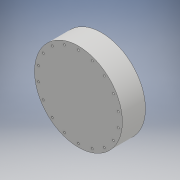
# Autodesk Inventor part: Korbbogenboden
Saved by Autodesk Inventor 2017 (Build 210142000, 142)
## iProperties
Created: 2019-06-21
Part Number: Korbbogenboden
Material: Generic
Document SubType Name: Modeling
Designer: Ole Simmering
Density: 1 g/cm^3
Appearance: Default
Author: Ole Simmering
Autodesk Inventor part; units mm, degrees
ref_plane "YZ Plane" through (0, 0, 0) normal (1, 0, 0) x (0, 1, 0)
ref_plane "XZ Plane" through (0, 0, 0) normal (0, 1, 0) x (-1, 0, 0)
ref_plane "XY Plane" through (0, 0, 0) normal (0, 0, 1) x (1, 0, 0)
sketch "Sketch1" plane through (0, 0, 0) normal (0, 0, 1) x (1, 0, 0)
  line L0 (0, 26.4298) -> (0, -158.7692) construction
  line L1 (144, 0) -> (144, -25)
  arc A0 (125.4705, -49.1481) -> (144, -25) centre (119, -25) ccw
  arc A1 (0, -66.1697) -> (125.4705, -49.1481) centre (-3.939, 433.8148) ccw
  line L2 (144, 0) -> (190, 0)
  line L3 (190, 0) -> (190, -100)
  line L4 (190, -100) -> (0, -100)
  line L5 (144, -25) -> (119, -25) construction
  line L6 (125.4705, -49.1481) -> (119, -25) construction
  line L7 (0, -66.1697) -> (0, -100)
  point P0 (0, 0)
  dimension "d0" = 288
  dimension "d1" = 380
  dimension "d2" = 100
  dimension "d3" = 25
  dimension "d4" = 500
  dimension "d5" = 25
  dimension "d6" = 75
  constraints: 16 end point, 4 point on circle, 3 horizontal, 3 point on line, 2 centre point, 2 tangent, 2 vertical, 1 collinear, 1 midpoint, 1 perpendicular
  measures "d0" diameter of L1 L0
  measures "d1" diameter of L3 L0
  measures "d2" distance of L2.end L3.end
  measures "d3" radius of A0
  measures "d4" radius of A1
  measures "d5" distance of L1.start L1.end
  measures "d6" angle of L6 L5
revolve "Revolution1" add sketch "Sketch1" angle 360 about axis through (0, 26.4298, 0) along (0, -1, 0)
sketch "Sketch2" plane through (0, 0, 0) normal (0, 1, 0) x (1, 0, 0)
  point P0 (0, 0)
  point P1 (0, -175)
  point P2 (0, 0)
  dimension "d8" = 175
  constraints: 1 coincident
  measures "d8" distance of point (0, 0) point (0, -175)
hole "Hole1" at (0, 0, 175) direction (0, -1, 0) diameter 8.376 end through all thread size "M10x1.5" class "6H" standard "ISO Metric profile"
pattern_circular "Circular Pattern1" count 18 over 360 about axis through (0, -12.5, 0) along (0, -1, 0) of "Hole1"
body "Solid1"
